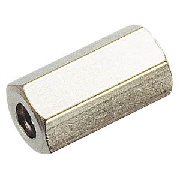
# Autodesk Inventor part: Diszanzbolzen_M4x20
Saved by Autodesk Inventor 2016 (Build 200138000, 138)
## iProperties
Created: 2012-04-06
Part Number: Diszanzbolzen_M4x20
Document SubType Name: Modeling
Designer: 4ndreas
Density: 8.83 g/cm^3
Mass: 5.93457 g
Surface Area: 7.33461 cm^2
Volume: 0.672091 cm^3
Material: Nickel-Kupfer-Legierung 400
Appearance: Chrom - poliert
Author: 4ndreas
Autodesk Inventor part; units mm, degrees
ref_plane "YZ Plane" through (0, 0, 0) normal (1, 0, 0) x (0, 1, 0)
ref_plane "XZ Plane" through (0, 0, 0) normal (0, 1, 0) x (-1, 0, 0)
ref_plane "XY Plane" through (0, 0, 0) normal (0, 0, 1) x (1, 0, 0)
sketch "Skizze1" plane through (0, 0, 0) normal (0, 0, 1) x (1, 0, 0)
  line L0 (4.0415, 0) -> (2.0207, -3.5)
  line L1 (2.0207, -3.5) -> (-2.0207, -3.5)
  line L2 (-2.0207, -3.5) -> (-4.0415, 0)
  line L3 (-4.0415, 0) -> (-2.0207, 3.5)
  line L4 (-2.0207, 3.5) -> (2.0207, 3.5)
  line L5 (2.0207, 3.5) -> (4.0415, 0)
  point P0 (0, 0)
  point P1 (0, 0)
  dimension "d0" = 7
  constraints: 12 end point, 1 coincident, 13 other
  measures "d0" distance between parallel lines of L1 L4
extrude "Extrusion1" add sketch "Skizze1" along normal blind 20
sketch "Skizze2" plane through (0, 0, 20) normal (0, 0, 1) x (1, 0, 0)
  point P0 (0, 0)
hole "Bohrung1" at (0, 0, 20) direction (0, 0, -1) diameter 3.242 end through all thread size "M4x0.7" class "6H" standard "ISO Metric profile"
chamfer "Fase2" distance 0.7 angle 45 12 edges at (3.0311, -1.75, 20) (0, -3.5, 20) (-3.0311, -1.75, 20) (-3.0311, 1.75, 20) (0, 3.5, 20) (3.0311, 1.75, 20) (0, -3.5, 0) (3.0311, -1.75, 0) (3.0311, 1.75, 0) (0, 3.5, 0) (-3.0311, 1.75, 0) (-3.0311, -1.75, 0)
chamfer "Fase3" distance 0.2 angle 45 2 edges at (0, 1.621, 20) (0, 1.621, 0)
